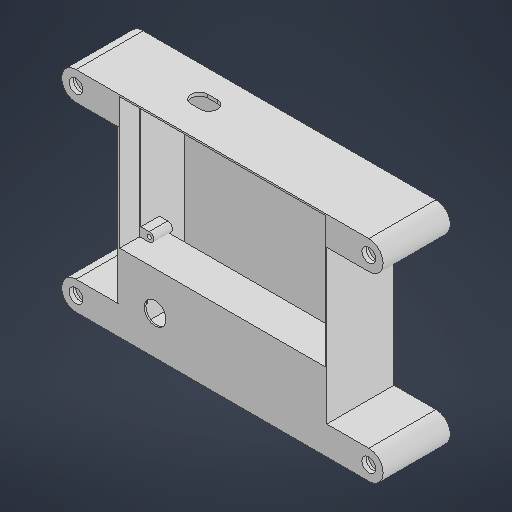
# Autodesk Inventor part: door-opener-v2-enclosure
Saved by Autodesk Inventor 2026.1 (Build 301233020, 233B)
## iProperties
Created: 2025-11-21
Part Number: door-opener-v2-enclosure
Material: Generic
Document SubType Name: Modeling
Designer: ericswpark
Density: 1 g/cm^3
Appearance: Default
Author: ericswpark
Autodesk Inventor part; units mm, degrees
ref_plane "YZ Plane" through (0, 0, 0) normal (1, 0, 0) x (0, 1, 0)
ref_plane "XZ Plane" through (0, 0, 0) normal (0, 1, 0) x (-1, 0, 0)
ref_plane "XY Plane" through (0, 0, 0) normal (0, 0, 1) x (1, 0, 0)
sketch "Sketch1" plane through (0, 0, 0) normal (0, 0, 1) x (1, 0, 0)
  line L0 (0, 0) -> (124.3, 0)
  line L1 (124.3, 0) -> (124.3, 125.1)
  line L2 (124.3, 125.1) -> (0, 125.1)
  line L3 (0, 125.1) -> (0, 0)
  circle A0 centre (149.3, 116.6) radius 8.5
  line L4 (124.3, 125.1) -> (149.3, 125.1)
  line L5 (149.3, 125.1) -> (149.3, 108.1)
  line L6 (149.3, 108.1) -> (124.3, 108.1)
  line L7 (124.3, 108.1) -> (124.3, 125.1)
  circle A1 centre (149.3, 116.6) radius 5.675
  circle A2 centre (-25, 116.6) radius 5.675
  circle A3 centre (-25, 116.6) radius 8.5
  line L8 (-25, 108.1) -> (0, 108.1)
  line L9 (0, 108.1) -> (0, 125.1)
  line L10 (0, 125.1) -> (-25, 125.1)
  line L11 (-25, 125.1) -> (-25, 108.1)
  circle A4 centre (149.3, 8.5) radius 5.675
  circle A5 centre (149.3, 8.5) radius 8.5
  line L12 (149.3, 17) -> (124.3, 17)
  line L13 (124.3, 17) -> (124.3, 0)
  line L14 (124.3, 0) -> (149.3, 0)
  line L15 (149.3, 0) -> (149.3, 17)
  line L16 (0, 17) -> (-25, 17)
  line L17 (-25, 17) -> (-25, 0)
  line L18 (-25, 0) -> (0, 0)
  line L19 (0, 0) -> (0, 17)
  circle A6 centre (-25, 8.5) radius 5.675
  circle A7 centre (-25, 8.5) radius 8.5
  point P0 (0, 108.1)
  dimension "d0" = 124.3
  dimension "d1" = 125.1
  dimension "d87" = 25
  dimension "d88" = 17
  dimension "d89" = 11.35
  dimension "d90" = 11.35
  dimension "d91" = 17
  dimension "d92" = 25
  dimension "d93" = 11.35
  dimension "d94" = 17
  dimension "d95" = 25
  dimension "d96" = 11.35
  dimension "d97" = 17
  dimension "d98" = 25
  constraints: 40 end point, 10 parallel, 8 centre point, 8 tangent, 6 midpoint, 5 horizontal, 5 perpendicular, 4 coincident, 3 point on line
  measures "d0" distance between parallel lines of L1 L3
  measures "d1" distance between parallel lines of L0 L2
  measures "d87" distance from line of L1 point (149.3, 116.6)
  measures "d88" diameter of A0
  measures "d89" diameter of A1
  measures "d90" diameter of A2
  measures "d91" diameter of A3
  measures "d92" distance from line of L3 point (-25, 116.6)
  measures "d93" diameter of A6
  measures "d94" diameter of A7
  measures "d95" distance from line of L3 A6.centre
  measures "d96" diameter of A4
  measures "d97" diameter of A5
  measures "d98" distance from line of L1 A4.centre
extrude "Extrusion1" add sketch "Sketch1" along normal blind 40
sketch "Sketch2" plane through (0, 0, 0) normal (0, 0, -1) x (-1, 0, 0)
  line L0 (0, 0) -> (-124.3, 0) projected
  line L1 (-2, 0) -> (-122.3, 0)
  line L2 (-122.3, 0) -> (-122.3, 123.1)
  line L3 (-122.3, 123.1) -> (-2, 123.1)
  line L4 (-2, 123.1) -> (-2, 0)
  line L5 (0, 108.1) -> (0, 0) projected
  line L6 (-124.3, 17) -> (-124.3, 108.1) projected
  line L7 (-124.3, 125.1) -> (0, 125.1) projected
  point P0 (-122.3, 0)
  dimension "d4" = 2
  dimension "d5" = 2
  dimension "d6" = 2
  constraints: 8 end point, 2 parallel, 1 horizontal, 1 perpendicular, 1 point on line
  measures "d4" distance between parallel lines of L5 L4
  measures "d5" distance between parallel lines of L2 L6
  measures "d6" distance between parallel lines of L7 L3
extrude "Extrusion2" cut sketch "Sketch2" against normal blind 1
sketch "Sketch3" plane through (0, 0, 40) normal (0, -1, 0) x (1, 0, 0)
  line L0 (123.3, -39) -> (1, -39)
  line L1 (1, -39) -> (1, -37.5)
  line L2 (1, -37.5) -> (123.3, -37.5)
  line L3 (123.3, -37.5) -> (123.3, -39)
  line L4 (2, -39) -> (122.3, -39) projected
  line L5 (0, -40) -> (0, 0) projected
  line L6 (124.3, -40) -> (124.3, 0) projected
  dimension "d9" = 1
  dimension "d10" = 1
  dimension "d11" = 1.5
  constraints: 8 end point, 2 parallel, 1 collinear, 1 horizontal, 1 perpendicular
  measures "d9" distance between parallel lines of L5 L1
  measures "d10" distance between parallel lines of L6 L3
  measures "d11" distance between parallel lines of L0 L2
extrude "Extrusion3" cut sketch "Sketch3" against normal blind 124.1
sketch "Sketch4" plane through (123.3, 0, 2.5) normal (0, 0, -1) x (-1, 0, 0)
  line L0 (121.3, 1) -> (1, 1)
  line L1 (1, 1) -> (1, 123.1)
  line L2 (1, 123.1) -> (121.3, 123.1)
  line L3 (121.3, 123.1) -> (121.3, 1)
  line L4 (122.3, 0) -> (0, 0) projected
  line L5 (0, 0) -> (0, 124.1) projected
  line L6 (122.3, 0) -> (122.3, 124.1) projected
  line L7 (122.3, 124.1) -> (0, 124.1) projected
  point P0 (123.3, 0)
  dimension "d14" = 1
  dimension "d15" = 1
  dimension "d16" = 1
  dimension "d17" = 1
  constraints: 8 end point, 2 parallel, 1 horizontal, 1 perpendicular
  measures "d14" distance between parallel lines of L4 L0
  measures "d15" distance between parallel lines of L1 L5
  measures "d16" distance between parallel lines of L6 L3
  measures "d17" distance between parallel lines of L2 L7
extrude "Extrusion4" cut sketch "Sketch4" against normal blind 36.5 contours L0 L1 L2 L3
sketch "Sketch6" plane through (123.3, 0, 39) normal (0, 0, -1) x (-1, 0, 0)
  circle A0 centre (6, 118.1) radius 2.75
  circle A1 centre (116.3, 118.1) radius 2.75
  circle A2 centre (116.3, 49) radius 2.75
  circle A3 centre (6, 49) radius 2.75
  line L0 (1, 123.1) -> (121.3, 123.1) projected
  line L1 (1, 1) -> (1, 123.1) projected
  line L2 (121.3, 123.1) -> (121.3, 1) projected
  line L3 (1, 0) -> (1, 123.1) projected
  line L4 (6, 46.25) -> (1, 46.25)
  line L5 (1, 46.25) -> (1, 51.75)
  line L6 (1, 51.75) -> (6, 51.75)
  line L7 (6, 51.75) -> (6, 46.25)
  line L8 (116.3, 51.75) -> (121.3, 51.75)
  line L9 (121.3, 51.75) -> (121.3, 46.25)
  line L10 (121.3, 46.25) -> (116.3, 46.25)
  line L11 (116.3, 46.25) -> (116.3, 51.75)
  line L12 (1, 123.1) -> (8.75, 123.1)
  line L13 (8.75, 123.1) -> (8.75, 115.35)
  line L14 (8.75, 115.35) -> (1, 115.35)
  line L15 (1, 115.35) -> (1, 123.1)
  line L16 (121.3, 123.1) -> (113.55, 123.1)
  line L17 (113.55, 123.1) -> (113.55, 115.35)
  line L18 (113.55, 115.35) -> (121.3, 115.35)
  line L19 (121.3, 115.35) -> (121.3, 123.1)
  circle A4 centre (6, 49) radius 1.25
  circle A5 centre (116.3, 49) radius 1.25
  circle A6 centre (116.3, 118.1) radius 1.25
  circle A7 centre (6, 118.1) radius 1.25
  point P0 (123.3, 0)
  point P1 (6, 51.75)
  point P2 (1, 51.75)
  point P3 (1, 46.25)
  point P4 (116.3, 46.25)
  point P5 (113.55, 118.1)
  point P6 (116.3, 115.35)
  point P7 (113.55, 123.1)
  point P8 (6, 115.35)
  point P9 (8.75, 118.1)
  point P10 (8.75, 123.1)
  point P11 (1, 115.35)
  dimension "d36" = 5.5
  dimension "d37" = 5.5
  dimension "d26" = 5
  dimension "d27" = 5
  dimension "d28" = 5
  dimension "d29" = 5
  dimension "d30" = 5
  dimension "d31" = 5
  dimension "d32" = 74.1
  dimension "d33" = 74.1
  dimension "d34" = 5.5
  dimension "d35" = 5.5
  dimension "d46" = 2.5
  dimension "d47" = 2.5
  dimension "d48" = 2.5
  dimension "d49" = 2.5
  constraints: 32 end point, 8 parallel, 7 horizontal, 6 centre point, 4 coincident, 4 perpendicular, 4 tangent, 1 collinear, 1 midpoint, 1 point on line, 6 other
  measures "d26" distance from line of L0 A0.centre
  measures "d27" distance from line of L1 A0.centre
  measures "d28" distance from line of L0 A1.centre
  measures "d29" distance from line of L2 A1.centre
  measures "d30" distance from line of L2 point (116.3, 49)
  measures "d31" distance from line of L3 point (6, 49)
  measures "d32" distance from line of L0 point (6, 49)
  measures "d33" distance from line of L0 point (116.3, 49)
  measures "d34" diameter of A0
  measures "d35" diameter of A1
  measures "d46" diameter of A4
  measures "d47" diameter of A5
  measures "d48" diameter of A6
  measures "d49" diameter of A7
extrude "Extrusion6" add sketch "Sketch6" along normal blind 21.6 contours A0 | A0 L14 L1 L0 L13 | A1 | A1 L17 L0 L2 L18 | A2 L11 A5 | A2 L8 L2 L10 | L11 A5 A2 | A3 L7 A4 | L7 A4 A3 | A3 L4 L1 L6
sketch "Sketch7" plane through (0, 0, 40) normal (0, 0, 1) x (1, 0, 0)
  line L0 (1, 124.1) -> (123.3, 124.1)
  line L1 (123.3, 124.1) -> (123.3, 46)
  line L2 (123.3, 46) -> (1, 46)
  line L3 (1, 46) -> (1, 124.1)
  line L4 (0, 108.1) -> (0, 0) projected
  line L5 (124.3, 125.1) -> (0, 125.1) projected
  line L6 (124.3, 17) -> (124.3, 108.1) projected
  point P0 (124.3, 0)
  dimension "d40" = 1
  dimension "d41" = 1
  dimension "d42" = 1
  dimension "d43" = 78.1
  constraints: 8 end point, 2 parallel, 1 horizontal, 1 perpendicular
  measures "d40" distance between parallel lines of L4 L3
  measures "d41" distance between parallel lines of L5 L0
  measures "d42" distance between parallel lines of L6 L1
  measures "d43" distance between parallel lines of L0 L2
extrude "Extrusion7" cut sketch "Sketch7" against normal blind 11.6
sketch "Sketch9" plane through (123.3, 0, 39) normal (0, 0, -1) x (-1, 0, 0)
  line L0 (1, 1) -> (1, 46) projected
  line L1 (121.3, 46) -> (121.3, 1) projected
  line L2 (1, 46) -> (121.3, 46)
  line L3 (121.3, 46) -> (121.3, 44)
  line L4 (121.3, 44) -> (1, 44)
  line L5 (1, 44) -> (1, 46)
  point P0 (123.3, 0)
  point P1 (121.3, 46)
  point P2 (1, 44)
  dimension "d50" = 2
  constraints: 8 end point, 2 parallel, 1 horizontal, 1 perpendicular, 1 point on line
  measures "d50" distance between parallel lines of L2 L4
extrude "Extrusion8" add sketch "Sketch9" along normal blind 21.5
sketch "Sketch10" plane through (123.3, 0, 39) normal (0, 0, -1) x (-1, 0, 0)
  circle A0 centre (9, 36) radius 2.25
  circle A1 centre (37, 10) radius 2.25
  circle A2 centre (37, 10) radius 3.25
  circle A3 centre (9, 36) radius 3.25
  line L0 (121.3, 44) -> (1, 44) projected
  line L1 (1, 1) -> (1, 44) projected
  point P0 (123.3, 0)
  dimension "d53" = 4.5
  dimension "d54" = 6.5
  dimension "d55" = 8
  dimension "d56" = 8
  dimension "d57" = 4.5
  dimension "d58" = 6.5
  dimension "d59" = 28
  dimension "d60" = 26
  constraints: 4 centre point, 2 coincident
  measures "d53" diameter of A0
  measures "d54" diameter of A3
  measures "d55" distance from line of A0.centre L0
  measures "d56" distance from line of L1 A0.centre
  measures "d57" diameter of A1
  measures "d58" diameter of A2
  measures "d59" horizontal distance of A0.centre A1.centre
  measures "d60" vertical distance of A0.centre A1.centre
extrude "Extrusion9" add sketch "Sketch10" along normal blind 3
sketch "Sketch11" plane through (123.3, 0, 39) normal (0, 0, -1) x (-1, 0, 0)
  circle A0 centre (111.3, 11) radius 1.6
  circle A1 centre (111.3, 11) radius 2.1
  circle A2 centre (91.1, 11) radius 1.6
  circle A3 centre (91.1, 11) radius 2.1
  circle A4 centre (111.3, 23) radius 1.6
  circle A5 centre (111.3, 23) radius 2.1
  circle A6 centre (91.1, 23) radius 1.6
  circle A7 centre (91.1, 23) radius 2.1
  line L0 (121.3, 44) -> (121.3, 1) projected
  line L1 (121.3, 1) -> (1, 1) projected
  circle A8 centre (101.2, 23) radius 6.5
  line L2 (91.1, 23) -> (111.3, 23)
  point P0 (123.3, 0)
  dimension "d63" = 3.2
  dimension "d64" = 4.2
  dimension "d65" = 3.2
  dimension "d66" = 4.2
  dimension "d67" = 4.2
  dimension "d68" = 4.2
  dimension "d69" = 3.2
  dimension "d70" = 3.2
  dimension "d72" = 20.2
  dimension "d73" = 12
  dimension "d74" = 20.2
  dimension "d75" = 12
  dimension "d76" = 0
  dimension "d77" = 0
  dimension "d78" = 10
  dimension "d79" = 10
  dimension "d82" = 10.1
  dimension "d83" = 0
  dimension "d84" = 13
  constraints: 9 centre point, 4 coincident, 2 end point
  measures "d63" diameter of A6
  measures "d64" diameter of A7
  measures "d65" diameter of A4
  measures "d66" diameter of A5
  measures "d67" diameter of A3
  measures "d68" diameter of A1
  measures "d69" diameter of A2
  measures "d70" diameter of A0
  measures "d72" distance of A4.centre A6.centre
  measures "d73" distance of A0.centre A4.centre
  measures "d74" distance of A2.centre A0.centre
  measures "d75" distance of A6.centre A2.centre
  measures "d76" horizontal distance of A2.centre A6.centre
  measures "d77" vertical distance of A6.centre A4.centre
  measures "d78" distance from line of L0 A1.centre
  measures "d79" distance from line of L1 A0.centre
  measures "d82" distance of A8.centre A6.centre
  measures "d83" vertical distance of A6.centre A8.centre
  measures "d84" diameter of A8
extrude "Extrusion10" add sketch "Sketch11" along normal blind 2.5 contours A1 | A3 | A5 | A7
extrude "Extrusion11" cut sketch "Sketch11" against normal blind 1 contours L2 A8 | A8 L2
sketch "Sketch13" plane through (0, 0, 40) normal (0, 0, 1) x (1, 0, 0)
  circle A0 centre (-25, 116.6) radius 4.1
  circle A1 centre (-25, 8.5) radius 4.1
  circle A2 centre (149.3, 8.5) radius 4.1
  circle A3 centre (149.3, 116.6) radius 4.1
  line L0 (123.3, 124.1) -> (123.3, 46) projected
  line L1 (124.3, 108.1) -> (149.3, 108.1) projected
  line L2 (1, 46) -> (1, 124.1) projected
  line L3 (-25, 108.1) -> (0, 108.1) projected
  line L4 (149.3, 17) -> (124.3, 17) projected
  line L5 (124.3, 17) -> (124.3, 108.1) projected
  line L6 (0, 108.1) -> (0, 17) projected
  line L7 (0, 17) -> (-25, 17) projected
  point P0 (0, 0)
  dimension "d126" = 8.2
  dimension "d127" = 8.5
  dimension "d128" = 8.2
  dimension "d130" = 8.5
  dimension "d131" = 8.5
  dimension "d132" = 8.2
  dimension "d133" = 25
  dimension "d134" = 25
  dimension "d135" = 25
  dimension "d136" = 25
  dimension "d137" = 8.2
  dimension "d138" = 8.5
  constraints: 4 centre point
  measures "d126" diameter of A3
  measures "d127" distance from line of L1 A3.centre
  measures "d128" diameter of A0
  measures "d130" distance from line of L3 A0.centre
  measures "d131" distance from line of L4 A2.centre
  measures "d132" diameter of A2
  measures "d133" distance from line of L5 A2.centre
  measures "d134" distance from line of L5 A3.centre
  measures "d135" distance from line of L6 A0.centre
  measures "d136" distance from line of L6 A1.centre
  measures "d137" diameter of A1
  measures "d138" distance from line of L7 A1.centre
extrude "Extrusion12" cut sketch "Sketch13" against normal blind 6.3
ref_plane "Work Plane1" through (0, 0, 37.5) normal (0, 0, 1) x (1, 0, 0)
sketch "Sketch14" plane through (0, 0, 37.5) normal (0, 0, 1) x (1, 0, 0)
  circle A0 centre (-25, 116.6) radius 4.1 projected
  circle A1 centre (-25, 116.6) radius 7.25
  circle A2 centre (149.3, 116.6) radius 4.1 projected
  circle A3 centre (149.3, 116.6) radius 7.25
  circle A4 centre (149.3, 8.5) radius 4.1 projected
  circle A5 centre (149.3, 8.5) radius 7.25
  circle A6 centre (-25, 8.5) radius 4.1 projected
  circle A7 centre (-25, 8.5) radius 7.25
  point P0 (0, 0)
  dimension "d142" = 14.5
  dimension "d143" = 14.5
  dimension "d144" = 14.5
  dimension "d145" = 14.5
  constraints: 4 centre point, 4 coincident
  measures "d142" diameter of A1
  measures "d143" diameter of A7
  measures "d144" diameter of A5
  measures "d145" diameter of A3
extrude "Suction cup inner nub cut" cut sketch "Sketch14" against normal blind 3.8
sketch "Sketch16" plane through (0, 124.1, 40) normal (0, -1, 0) x (1, 0, 0)
  line L0 (123.3, -37.5) -> (123.3, -39) projected
  line L1 (1, -39) -> (1, -37.5) projected
  line L2 (123.3, -37.5) -> (1, -37.5)
  line L3 (1, -37.5) -> (1, -39)
  line L4 (1, -39) -> (123.3, -39)
  line L5 (123.3, -39) -> (123.3, -37.5)
  point P0 (0, -40)
  constraints: 8 end point, 2 parallel, 1 horizontal, 1 perpendicular
extrude "BackPlate inner" add sketch "Sketch16" along normal blind 124.1 separate body
sketch "Sketch17" plane through (123.3, 124.1, 1) normal (0, 0, -1) x (-1, 0, 0)
  line L0 (122.3, -124.1) -> (0, -124.1) projected
  line L1 (121.3, -124.1) -> (1, -124.1)
  line L2 (1, -124.1) -> (1, -1)
  line L3 (1, -1) -> (121.3, -1)
  line L4 (121.3, -1) -> (121.3, -124.1)
  line L5 (1, -1) -> (121.3, -1) projected
  line L6 (1, -124.1) -> (1, -1) projected
  line L7 (121.3, -1) -> (121.3, -124.1) projected
  point P0 (123.3, -124.1)
  point P1 (1, -124.1)
  constraints: 8 end point, 3 collinear, 2 parallel, 1 horizontal, 1 perpendicular, 1 point on line
extrude "BackPlate outer" add sketch "Sketch17" along normal blind 1 bodies 2
sketch "Sketch19" plane through (2, 123.1, 2.5) normal (0, -1, 0) x (1, 0, 0)
  line L0 (25, 16) -> (30.5, 16) construction
  line L1 (25, 11) -> (30.5, 11)
  line L2 (30.5, 21) -> (25, 21)
  arc A0 (25, 21) -> (25, 11) centre (25, 16) ccw
  arc A1 (30.5, 11) -> (30.5, 21) centre (30.5, 16) ccw
  line L3 (-1, 37.5) -> (121.3, 37.5) projected
  point P0 (-2, -2.5)
  point P1 (27.75, 16)
  point P2 (20, 16)
  point P3 (35.5, 16)
  dimension "d156" = 16.5
  dimension "d157" = 21
  dimension "d158" = 10
  dimension "d159" = 15.5
  constraints: 8 end point, 6 point on circle, 4 tangent, 2 centre point, 1 horizontal, 1 midpoint, 1 parallel
  measures "d156" distance between parallel lines of L2 L3
  measures "d157" horizontal distance of point (20, 16) L3.start
  measures "d158" distance between parallel lines of L1 L2
  measures "d159" distance of point (35.5, 16) point (20, 16)
extrude "USB-C cutout" cut sketch "Sketch19" against normal blind 5 bodies 1
sketch "Sketch20" plane through (123.3, 0, 39) normal (0, 0, -1) x (-1, 0, 0)
  circle A0 centre (61.15, 6.25) radius 2.25
  circle A1 centre (61.15, 6.25) radius 3.25
  line L0 (121.3, 1) -> (1, 1) projected
  line L1 (1, 1) -> (1, 44) projected
  line L2 (121.3, 44) -> (121.3, 1) projected
  line L3 (64.4, 1) -> (57.9, 1)
  line L4 (57.9, 1) -> (57.9, 6.25)
  line L5 (57.9, 6.25) -> (64.4, 6.25)
  line L6 (64.4, 6.25) -> (64.4, 1)
  point P0 (123.3, 0)
  point P1 (64.4, 6.25)
  point P2 (57.9, 6.25)
  point P3 (57.9, 1)
  dimension "d162" = 4.5
  dimension "d163" = 6.5
  dimension "d165" = 2
  dimension "d166" = 60.15
  dimension "d167" = 60.15
  constraints: 8 end point, 2 centre point, 2 parallel, 2 tangent, 1 coincident, 1 horizontal, 1 midpoint, 1 perpendicular, 1 point on line
  measures "d162" diameter of A0
  measures "d163" diameter of A1
  measures "d165" distance edge to line of A1 L0
  measures "d166" distance from line of L1 A0.centre
  measures "d167" distance from line of L2 A0.centre
extrude "Extrusion17" add sketch "Sketch20" along normal blind 22 contours L5 A1 A0 | A0 L5 A1 | L6 L0 L4 A1 bodies 1
sketch "Sketch22" plane through (62.15, 6.25, 39) normal (0, 0, -1) x (-1, 0, 0)
  circle A0 centre (0, 0) radius 2.25 projected
  circle A1 centre (0, 0) radius 2.25
  point P0 (62.15, -6.25)
  constraints: 1 centre point, 1 coincident, 1 concentric
extrude "Extrusion18" add sketch "Sketch22" along normal blind 19 bodies 1
sketch "Sketch23" plane through (123.3, 124.1, 0) normal (0, 0, -1) x (-1, 0, 0)
  circle A0 centre (61.15, -117.85) radius 2.25
  line L0 (1, -124.1) -> (121.3, -124.1) projected
  line L1 (121.3, -123.1) -> (1, -123.1) projected
  line L2 (1, -124.1) -> (1, -1) projected
  point P0 (123.3, -124.1)
  dimension "d172" = 4.5
  dimension "d174" = 3
  dimension "d175" = 60.15
  constraints: 1 centre point
  measures "d172" diameter of A0
  measures "d174" distance edge to line of A0 L1
  measures "d175" distance from line of L2 A0.centre
extrude "Extrusion19" cut sketch "Sketch23" against normal blind 2.5 bodies 2
equation "\"d0\" = enclosure_total_width"
equation "\"d1\" = enclosure_total_height"
equation "\"d2\" = enclosure_thickness"
equation "\"d4\" = 2 * wall_thickness"
equation "\"d5\" = 2 * wall_thickness"
equation "\"d6\" = 2 * wall_thickness"
equation "\"d7\" = enclosure_back_and_plate_distance"
equation "\"d9\" = wall_thickness"
equation "\"d10\" = wall_thickness"
equation "\"d11\" = enclosure_back_plate_thickness"
equation "\"d12\" = enclosure_total_height - wall_thickness"
equation "\"d14\" = wall_thickness"
equation "\"d15\" = wall_thickness"
equation "\"d16\" = wall_thickness"
equation "\"d17\" = wall_thickness"
equation "\"d18\" = enclosure_thickness - 2 * wall_thickness - enclosure_back_plate_thickness"
equation "\"d36\" = rpi_screen_screw_post_diameter"
equation "\"d37\" = rpi_screen_screw_post_diameter"
equation "\"d26\" = rpi_screen_screw_hole_side_distance + tolerances"
equation "\"d27\" = rpi_screen_screw_hole_side_distance + tolerances"
equation "\"d28\" = rpi_screen_screw_hole_side_distance + tolerances"
equation "\"d29\" = rpi_screen_screw_hole_side_distance + tolerances"
equation "\"d30\" = rpi_screen_screw_hole_side_distance + tolerances"
equation "\"d31\" = rpi_screen_screw_hole_side_distance + tolerances"
equation "\"d32\" = -rpi_screen_screw_hole_side_distance + rpi_screen_height + tolerances"
equation "\"d33\" = -rpi_screen_screw_hole_side_distance + rpi_screen_height + tolerances"
equation "\"d34\" = rpi_screen_screw_post_diameter"
equation "\"d35\" = rpi_screen_screw_post_diameter"
equation "\"d38\" = rpi_screen_screw_post_depth + rpi_screen_screw_resting_plate_thickness"
equation "\"d40\" = wall_thickness"
equation "\"d41\" = wall_thickness"
equation "\"d42\" = wall_thickness"
equation "\"d43\" = rpi_screen_height"
equation "\"d44\" = rpi_screen_screw_post_depth"
equation "\"d50\" = separator_wall_between_rpi_and_modules"
equation "\"d53\" = nfc_module_standoff_inner_diameter"
equation "\"d54\" = nfc_module_standoff_inner_diameter + nfc_module_standoff_thickness"
equation "\"d55\" = nfc_module_screw_hole_side_distance + tolerances"
equation "\"d56\" = nfc_module_screw_hole_side_distance + tolerances"
equation "\"d57\" = nfc_module_standoff_inner_diameter"
equation "\"d58\" = nfc_module_standoff_inner_diameter + nfc_module_standoff_thickness"
equation "\"d59\" = nfc_module_width - 2 * nfc_module_screw_hole_side_distance"
equation "\"d60\" = nfc_module_height - 2 * nfc_module_screw_hole_side_distance"
equation "\"d61\" = nfc_module_standoff_depth"
equation "\"d63\" = rpi_camera_standoff_inner_diameter"
equation "\"d64\" = rpi_camera_standoff_inner_diameter + rpi_camera_standoff_thickness"
equation "\"d65\" = rpi_camera_standoff_inner_diameter"
equation "\"d66\" = rpi_camera_standoff_inner_diameter + rpi_camera_standoff_thickness"
equation "\"d67\" = rpi_camera_standoff_inner_diameter + rpi_camera_standoff_thickness"
equation "\"d68\" = rpi_camera_standoff_inner_diameter + rpi_camera_standoff_thickness"
equation "\"d69\" = rpi_camera_standoff_inner_diameter"
equation "\"d70\" = rpi_camera_standoff_inner_diameter"
equation "\"d72\" = rpi_camera_screw_hole_horizontal_apart"
equation "\"d73\" = rpi_camera_screw_hole_vertical_apart"
equation "\"d74\" = rpi_camera_screw_hole_horizontal_apart"
equation "\"d75\" = rpi_camera_screw_hole_vertical_apart"
equation "\"d78\" = rpi_camera_bottom_right_placement"
equation "\"d79\" = rpi_camera_bottom_right_placement"
equation "\"d80\" = rpi_camera_standoff_depth"
equation "\"rpi_screen_width\" = 121.3"
equation "\"rpi_screen_height\" = 78.1"
equation "\"rpi_screen_assembly_thickness\" = 32.8"
equation "\"tolerances\" = 0.5"
equation "\"wall_thickness\" = 1"
equation "\"rpi_camera_height\" = 24"
equation "\"rpi_camera_width\" = 25"
equation "\"rpi_camera_thickness\" = 12.7"
equation "\"nfc_module_height\" = 41"
equation "\"nfc_module_width\" = 43"
equation "\"nfc_module_screw_hole_side_distance\" = 7.5"
equation "\"nfc_module_screw_hole_diameter\" = 3"
equation "\"rpi_camera_screw_hole_diameter\" = 2"
equation "\"separator_wall_between_rpi_and_modules\" = 2"
equation "\"enclosure_total_height\" = 4 * tolerances + 2 * wall_thickness + rpi_screen_height + separator_wall_between_rpi_and_modules + nfc_module_height"
equation "\"enclosure_total_width\" = 2 * tolerances + 2 * wall_thickness + rpi_screen_width"
equation "\"enclosure_thickness\" = 40"
equation "\"enclosure_back_and_plate_distance\" = 1"
equation "\"enclosure_back_plate_thickness\" = 1.5"
equation "\"rpi_screen_screw_hole_diameter\" = 3"
equation "\"rpi_screen_screw_hole_side_distance\" = 4.5"
equation "\"rpi_screen_screw_post_depth\" = 11.6"
equation "\"rpi_screen_screw_post_diameter\" = 5.5"
equation "\"rpi_screen_screw_resting_plate_thickness\" = 10"
equation "\"nfc_module_standoff_inner_diameter\" = 4.5"
equation "\"rpi_camera_standoff_inner_diameter\" = 3.2"
equation "\"nfc_module_standoff_thickness\" = 2"
equation "\"rpi_camera_standoff_thickness\" = 1"
equation "\"nfc_module_standoff_depth\" = 3"
equation "\"rpi_camera_standoff_depth\" = 2.5"
equation "\"rpi_camera_screw_hole_vertical_apart\" = 12"
equation "\"rpi_camera_screw_hole_horizontal_apart\" = 20.2"
equation "\"rpi_camera_bottom_right_placement\" = 10"
equation "\"rpi_camera_hole_diameter\" = 13"
equation "\"suction_cup_distance_from_base\" = 25"
equation "\"suction_cup_inner_diameter\" = 8.2"
equation "\"suction_cup_nub_diameter\" = 14.5"
equation "\"suction_cup_arm_diameter\" = 17"
equation "\"suction_cup_inner_depth\" = 2.5"
equation "\"suction_cup_nub_depth\" = 3.8"
equation "\"usb_c_cutout_left_wall_distance\" = 21"
equation "\"usb_c_cutout_screen_distance\" = 16.5"
equation "\"usb_c_cutout_width\" = 15.5"
equation "\"back_plate_standoff_inner_diameter\" = 4.5"
equation "\"back_plate_standoff_thickness\" = 2"
equation "\"back_plate_standoff_depth\" = 22"
equation "\"back_plate_standoff_heat_set_insert_depth\" = 3"
equation "\"back_plate_standoff_from_bottom\" = 2"
